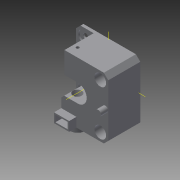
# Autodesk Inventor part: body
Saved by Autodesk Inventor 2014 (Build 180170000, 170)
## iProperties
Created: 2014-11-20
Part Number: body
Material: Generic
Document SubType Name: Modeling
Designer: KriMag
Density: 1 g/cm^3
Appearance: Default
Author: KriMag
Autodesk Inventor part; units mm, degrees
ref_plane "YZ Plane" through (0, 0, 0) normal (1, 0, 0) x (0, 1, 0)
ref_plane "XZ Plane" through (0, 0, 0) normal (0, 1, 0) x (-1, 0, 0)
ref_plane "XY Plane" through (0, 0, 0) normal (0, 0, 1) x (1, 0, 0)
sketch "Sketch1" plane through (0, 0, 0) normal (0, 1, 0) x (-1, 0, 0)
  line L0 (18, -21) -> (-18, -21)
  line L1 (-21, -18) -> (-21, 18)
  line L2 (-18, 21) -> (18, 21)
  line L3 (21, 18) -> (21, -18)
  line L4 (21, -21) -> (-21, 21) construction
  line L5 (-21, -21) -> (21, 21) construction
  line L6 (21, 18) -> (18, 21)
  line L7 (-21, -18) -> (-18, -21)
  line L8 (-18, 21) -> (-21, 18)
  line L9 (21, -18) -> (18, -21)
  line L10 (19.5, 19.5) -> (15.0999, 15.0999) construction
  circle A0 centre (15.5563, 15.5563) radius 1.75
  circle A1 centre (-15.5563, 15.5563) radius 1.75
  circle A2 centre (-15.5563, -15.5563) radius 1.75
  circle A3 centre (15.5563, -15.5563) radius 1.75
  circle A4 centre (0, 0) radius 6.25
  line L11 (-15.5563, 15.5563) -> (15.5563, -15.5563) construction
  dimension "d0" = 42
  dimension "d1" = 42
  dimension "d2" = 3
  dimension "d3" = 3
  dimension "d4" = 3
  dimension "d5" = 3
  dimension "d6" = 3
  dimension "d7" = 3
  dimension "d8" = 3
  dimension "d9" = 3
  dimension "d11" = 3.5
  dimension "d14" = 360
  dimension "d16" = 12.5
  dimension "d20" = 22
  constraints: 24 end point, 8 point on line, 5 centre point, 3 midpoint, 2 parallel, 1 coincident, 1 collinear, 1 horizontal, 1 perpendicular, 9 other
  measures "d0" distance of L4.end L5.end
  measures "d1" distance of L5.start L4.end
  measures "d2" distance of L3.start L5.end
  measures "d3" distance of L2.end L5.end
  measures "d4" distance of L1.start L5.start
  measures "d5" distance of L0.end L5.start
  measures "d6" distance of L2.start L4.end
  measures "d7" distance of L1.end L4.end
  measures "d8" distance of L3.end L4.start
  measures "d9" distance of L0.start L4.start
  measures "d11" diameter of A0
  measures "d16" diameter of A4
  measures "d20" distance of A0.centre point (0, 0)
extrude "Extrusion1" add sketch "Sketch1" along normal blind 1
sketch "Sketch3" plane through (0, 0, 0) normal (0, -1, 0) x (1, 0, 0)
  circle A0 centre (0, 0) radius 6.25 projected
  circle A1 centre (-15.5563, 15.5563) radius 1.75 projected
  line L0 (-21, 18) -> (-18, 21) projected
  line L1 (-21, -18) -> (-21, 18) projected
  line L2 (-18, -21) -> (-21, -18) projected
  line L3 (18, -21) -> (-18, -21) projected
  line L4 (21, -18) -> (18, -21) projected
  line L5 (21, 18) -> (21, -18) projected
  line L6 (18, 21) -> (21, 18) projected
  line L7 (-18, 21) -> (18, 21) projected
  circle A2 centre (-15.5563, 15.5563) radius 4
  circle A3 centre (-15.5563, -15.5563) radius 4
  circle A4 centre (15.5563, -15.5563) radius 4
  circle A5 centre (15.5563, 15.5563) radius 4
  dimension "d28" = 8
  dimension "d31" = 360
  constraints: 4 centre point, 1 coincident, 9 other
  measures "d28" diameter of A2
extrude "Extrusion3" add sketch "Sketch3" along normal blind 1 contours L0 L7 L6 L5 L4 L3 L2 L1
sketch "Sketch4" plane through (0, -1, 0) normal (0, -1, 0) x (1, 0, 0)
  circle A0 centre (0, 0) radius 6.25 projected
  circle A1 centre (15.5563, 15.5563) radius 4 projected
  circle A2 centre (15.5563, -15.5563) radius 4 projected
  line L0 (-18, -21) -> (18, -21) projected
  line L1 (18, -21) -> (21, -18) projected
  line L2 (21, -18) -> (21, 18) projected
  line L3 (21, 18) -> (18, 21) projected
  line L4 (18, 21) -> (-18, 21) projected
  line L5 (-9, 6.25) -> (-9, 21)
  line L6 (-11.2, -6.25) -> (-11.2, -21)
  line L7 (-11.2, -6.25) -> (0, -6.25)
  line L8 (-9, 6.25) -> (0, 6.25)
  dimension "d38" = 14.75
  dimension "d39" = 32.2
  dimension "d40" = 30
  constraints: 8 end point, 4 perpendicular, 2 point on circle, 2 point on line, 1 tangent
  measures "d38" distance of L6.start L6.end
  measures "d39" distance between parallel lines of L6 L2
  measures "d40" distance between parallel lines of L5 L2
extrude "Extrusion4" add sketch "Sketch4" along normal blind 20 contours A0 L8 L5 L4 L3 L2 L1 L0 L6 L7
chamfer "Chamfer1" distance 2 angle 45 1 edges at (-11.2, -11, -6.25)
sketch "Sketch5" plane through (-18, 1, 21) normal (0, 0, 1) x (1, 0, 0)
  line L0 (36, -22) -> (36, 0) projected
  line L1 (0, 0) -> (36, 0) projected
  circle A0 centre (12, -16) radius 1
  point P0 (18, -1)
  dimension "d46" = 2
  dimension "d47" = 16
  dimension "d48" = 24
  constraints: 1 centre point
  measures "d46" diameter of A0
  measures "d47" distance from line of A0.centre L1
  measures "d48" distance from line of L0 A0.centre
extrude "Extrusion5" cut sketch "Sketch5" against normal blind 20
sketch "Sketch6" plane through (18, 1, -21) normal (0, 0, -1) x (-1, 0, 0)
  line L0 (0, 0) -> (36, 0) projected
  line L1 (0, -22) -> (0, 0) projected
  circle A0 centre (24, -16) radius 2.5
  line L2 (29.2, -2) -> (29.2, -22) projected
  line L3 (29.2, -22) -> (0, -22) projected
  point P0 (18, -1)
  dimension "d51" = 5
  dimension "d52" = 16
  dimension "d53" = 24
  dimension "d63" = 5.2
  dimension "d72" = 6
  constraints: 1 centre point
  measures "d51" diameter of A0
  measures "d52" distance from line of L0 A0.centre
  measures "d53" distance from line of A0.centre L1
  measures "d63" distance from line of A0.centre L2
  measures "d72" distance from line of L3 A0.centre
extrude "Extrusion6" cut sketch "Sketch6" against normal blind 6
sketch "Sketch7" plane through (0, -21, -6.25) normal (0, 0, 1) x (1, 0, 0)
  line L0 (-9.2, 0) -> (-9.2, 20) projected
  circle A0 centre (-6.2, 6) radius 3
  line L1 (-18, 22) -> (18, 22) projected
  point P0 (0, 21)
  dimension "d57" = 16
  dimension "d58" = 3
  constraints: 1 centre point, 1 tangent
  measures "d57" distance from line of L1 A0.centre
  measures "d58" distance from line of L0 A0.centre
sketch "Sketch8" plane through (-6, -15, -15) normal (0, 0, -1) x (-1, 0, 0)
  circle A0 centre (0, 0) radius 2.5 projected
  circle A1 centre (0, 0) radius 1
  point P0 (-6, 15)
  dimension "d56" = 2
  constraints: 1 centre point, 1 coincident
  measures "d56" diameter of A1
loft "Loft1" cut profiles "Sketch8", "Sketch7" contours A1 / all
sketch "Sketch9" plane through (0, -21, 0) normal (0, -1, 0) x (1, 0, 0)
  line L0 (-11.2, -8.25) -> (-11.2, -21) projected
  line L1 (-11.2, -21) -> (18, -21) projected
  line L2 (-10.2, -17.4) -> (-1.8, -17.4)
  line L3 (-1.8, -17.4) -> (-1.8, -20)
  line L4 (-1.8, -20) -> (-10.2, -20)
  line L5 (-10.2, -20) -> (-10.2, -17.4)
  dimension "d73" = 8.4
  dimension "d74" = 2.6
  dimension "d75" = 1
  dimension "d76" = 1
  constraints: 8 end point, 2 parallel, 1 horizontal, 1 perpendicular
  measures "d73" distance of L3.end L4.end
  measures "d74" distance of L2.end L3.end
  measures "d75" distance between parallel lines of L4 L1
  measures "d76" distance between parallel lines of L0 L5
extrude "Extrusion8" cut sketch "Sketch9" against normal blind 12
sketch "Sketch12" plane through (0, -21, 0) normal (0, -1, 0) x (1, 0, 0)
  line L0 (-10.2, -17.4) -> (-1.8, -17.4)
  line L1 (-1.8, -17.4) -> (-1.8, -15.6)
  line L2 (-1.8, -15.6) -> (-10.2, -15.6)
  line L3 (-10.2, -15.6) -> (-10.2, -17.4)
  line L4 (-1.8, -20) -> (-10.2, -20) projected
  dimension "d79" = 1.8
  constraints: 8 end point, 3 parallel, 1 horizontal, 1 perpendicular
  measures "d79" distance of L1.end L0.end
extrude "Extrusion9" cut sketch "Sketch12" against normal blind 0.5
sketch "Sketch13" plane through (0, -21, 0) normal (0, -1, 0) x (1, 0, 0)
  line L0 (-1.8, -15.6) -> (-1.8, -20) projected
  line L1 (-1.8, -20) -> (-10.2, -20) projected
  line L2 (-10.2, -20) -> (-10.2, -15.6) projected
  line L3 (-10.2, -15.6) -> (-1.8, -15.6) projected
  line L4 (-11.2, -8.25) -> (-11.2, -21)
  line L5 (-11.2, -21) -> (18, -21) projected
  line L6 (-11.2, -21) -> (-0.8, -21)
  line L7 (-0.8, -21) -> (-0.8, -14.6)
  line L8 (-0.8, -14.6) -> (-11.2, -14.6)
  line L9 (-11.2, -14.6) -> (-11.2, -21)
  dimension "d98" = 1
  dimension "d99" = 1
  constraints: 10 end point, 4 parallel, 1 horizontal, 1 perpendicular
  measures "d98" distance between parallel lines of L8 L3
  measures "d99" distance between parallel lines of L0 L7
extrude "Extrusion10" add sketch "Sketch13" along normal blind 5
sketch "Sketch14" plane through (0, -21, 0) normal (0, -1, 0) x (1, 0, 0)
  line L0 (21, -18) -> (21, 18) projected
  line L1 (18, 21) -> (-9, 21) projected
  circle A0 centre (19, 0) radius 2
  dimension "d88" = 2
  dimension "d89" = 21
  dimension "d90" = 4
  constraints: 1 centre point
  measures "d88" distance from line of L0 A0.centre
  measures "d89" distance from line of L1 A0.centre
  measures "d90" diameter of A0
extrude "Extrusion11" add sketch "Sketch14" along normal blind 5
sketch "Sketch21" plane through (18, 1, -21) normal (0, 0, -1) x (-1, 0, 0)
  circle A0 centre (24, -16) radius 2.5 projected
  line L0 (0, 0) -> (36, 0) projected
  line L1 (29.2, -2) -> (29.2, -27) projected
  line L2 (29.2, -16) -> (29.2, 0)
  line L3 (29.2, 0) -> (18.8, 0)
  line L4 (18.8, 0) -> (18.8, -16)
  arc A1 (18.8, -16) -> (29.2, -16) centre (24, -16) ccw
  point P0 (18, -1)
  constraints: 6 end point, 2 collinear, 2 point on circle, 1 centre point, 1 coincident, 1 parallel, 1 point on line, 1 tangent
extrude "Extrusion14" add sketch "Sketch21" along normal blind 5
equation "\"d3\" = d2"
equation "\"d5\" = d4"
equation "\"d7\" = d6"
equation "\"d9\" = d8"
body "Solid1"
